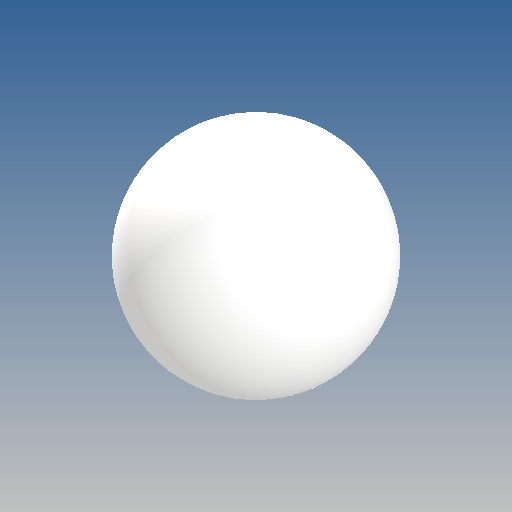
# Autodesk Inventor part: 52629-White
Saved by Autodesk Inventor 2025 (Build 290162010, 162A)
## iProperties
Created: 2024-11-23
Part Number: 52629-White
Material: ABS-Kunststoff
Document SubType Name: Modeling
Designer: hp.muther
Density: 1.06 g/cm^3
Appearance: White
Author: hp.muther
Autodesk Inventor part; units mm, degrees
ref_plane "YZ Plane" through (0, 0, 0) normal (1, 0, 0) x (0, 1, 0)
ref_plane "XZ Plane" through (0, 0, 0) normal (0, 1, 0) x (-1, 0, 0)
ref_plane "XY Plane" through (0, 0, 0) normal (0, 0, 1) x (1, 0, 0)
sketch "Skizze1" plane through (0, 0, 0) normal (0, 1, 0) x (-1, 0, 0)
  circle A0 centre (0, 0) radius 9.5
  line L0 (-9.2164, -2.3041) -> (9.2164, 2.3041)
  dimension "d0" = 19
  constraints: 2 end point, 2 point on circle, 1 centre point, 1 coincident, 1 midpoint
  measures "d0" diameter of A0
revolve "Umdrehung1" add sketch "Skizze1" angle 360 about axis through (9.2164, 0, -2.3041) along (-0.9701425, 0, 0.2425356) picked at (3.5648, -3.0616) contours A0 L0
